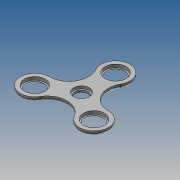
# Autodesk Inventor part: 014.004 Spinner
Saved by Autodesk Inventor 2016 SP1 (Build 200210100, 210)
## iProperties
Created: 2017-09-12
Part Number: 014.004 Spinner
Material: Stahl
Document SubType Name: Modeling
Density: 7.85 g/cm^3
Appearance: Stahl
Project: Fidget Spinner
Description: Spinner V2
Designer: BG
Mass: 29.7815 g
Surface Area: 37.272 cm^2
Volume: 3.79382 cm^3
Autodesk Inventor part; units mm, degrees
ref_plane "YZ Plane" through (0, 0, 0) normal (1, 0, 0) x (0, 1, 0)
ref_plane "XZ Plane" through (0, 0, 0) normal (0, 1, 0) x (-1, 0, 0)
ref_plane "XY Plane" through (0, 0, 0) normal (0, 0, 1) x (1, 0, 0)
sketch "Skizze2" plane through (0, 0, 0) normal (0, 0, 1) x (1, 0, 0)
  circle A0 centre (0, 0) radius 11
  circle A1 centre (0, 26) radius 11
  circle A2 centre (0, 26) radius 7
  line L0 (0, 6) -> (0, 0) construction
  line L1 (0, 0) -> (21.3014, 12.2984) construction
  line L2 (-18.5338, 10.7005) -> (0, 0) construction
  arc A3 (9.5263, 20.5) -> (9.5263, 5.5) centre (22.5167, 13) ccw
  arc A4 (-9.5263, 5.5) -> (-9.5263, 20.5) centre (-22.5167, 13) ccw
  dimension "d0" = 22
  dimension "d3" = 14
  dimension "d49" = 26
  dimension "d53" = 120
  dimension "d54" = 60
  constraints: 8 point on circle, 6 end point, 5 centre point, 4 tangent, 2 coincident, 2 point on line, 1 equal radius, 1 vertical, 1 vertical alignment
  measures "d0" diameter of A0
  measures "d3" diameter of A2
  measures "d49" distance of L0.end A2.centre
  measures "d53" angle of L2 L1
  measures "d54" angle of L1 L0
extrude "Extrusion1" add sketch "Skizze2" along normal blind 3.5
hole "Bohrung1" at (0, 26, 3.5) direction (0, 0, -1) diameter 16 depth 2.5
pattern_circular "Runde Anordnung2" count 3 over 360 about axis through (0, 0, 0) along (0, 0, 1) of "Extrusion1", "Bohrung1"
fillet "Rundung2" radius 2 3 edges at (0, 37, 0) (-32.0429, -18.5, 0) (32.0429, -18.5, 0)
fillet "Rundung2" radius 1 3 edges at (26.0167, -6.9378, 0) (-7, 26, 0) (-19.0167, -19.0622, 0)
sketch "Skizze3" plane through (0, 0, 0) normal (0, 0, -1) x (-1, 0, 0)
  point P0 (0, 0)
hole "Bohrung2" at (0, 0, 0) direction (0, 0, 1) diameter 10 end through all
hole "Bohrung3" at (0, 0, 3.5) direction (0, 0, -1) diameter 12 depth 2
